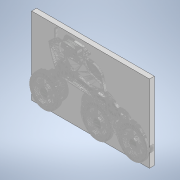
# Autodesk Inventor part: Rover 3 - Verde
Saved by Autodesk Inventor 2020.1 (Build 241239000, 239)
## iProperties
Created: 2020-06-20
Part Number: Rover 3 - Verde
Material: Genérico
Document SubType Name: Modeling
Designer: rotje
Density: 1 g/cm^3
Appearance: Valor por defecto
Author: rotje
Autodesk Inventor part; units mm, degrees
ref_plane "YZ Plane" through (0, 0, 0) normal (1, 0, 0) x (0, 1, 0)
ref_plane "XZ Plane" through (0, 0, 0) normal (0, 1, 0) x (-1, 0, 0)
ref_plane "XY Plane" through (0, 0, 0) normal (0, 0, 1) x (1, 0, 0)
sketch "Boceto1" plane through (28.317, 66.775, 0) normal (0, 0, -1) x (-1, 0, 0)
  line L0 (-122.0487, -64.2218) -> (28.317, -64.2218)
  line L1 (28.317, -64.2218) -> (28.317, 34.4982)
  line L2 (28.317, 34.4982) -> (-122.0487, 34.4982)
  line L3 (-122.0487, 34.4982) -> (-122.0487, -64.2218)
  point P0 (28.317, -66.775)
  constraints: 8 end point, 2 parallel, 1 horizontal, 1 perpendicular
extrude "Extrusión1" add sketch "Boceto1" along normal blind 1 and the other way blind 5.25
